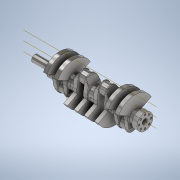
# Autodesk Inventor part: crankshaft
Saved by Autodesk Inventor 2021 (Build 250183000, 183)
## iProperties
Created: 2020-10-10
Part Number: crankshaft
Material: Сталь, высокопрочная, низколегированная
Document SubType Name: Modeling
Designer: panda
Density: 7.85 g/cm^3
Appearance: Сталь — полированная
Mass: 25968.1 g
Surface Area: 3777.36 cm^2
Volume: 3308.04 cm^3
Author: panda
Autodesk Inventor part; units mm, degrees
ref_plane "YZ Plane" through (0, 0, 0) normal (1, 0, 0) x (0, 1, 0)
ref_plane "XZ Plane" through (0, 0, 0) normal (0, 1, 0) x (-1, 0, 0)
ref_plane "XY Plane" through (0, 0, 0) normal (0, 0, 1) x (1, 0, 0)
sketch "Эскиз1" plane through (0, 0, 0) normal (1, 0, 0) x (0, 1, 0)
  circle A0 centre (0, 0) radius 27
  dimension "d0" = 54
  constraints: 1 centre point, 1 coincident
  measures "d0" diameter of A0
extrude "Выдавливание1" add sketch "Эскиз1" along normal blind 16.5
ref_plane "РабПлоскость1" through (36.5, 0, 0) normal (1, 0, 0) x (0, 0, -1)
sketch "Эскиз2" plane through (36.5, 0, 0) normal (1, 0, 0) x (0, 0, -1)
  circle A0 centre (0, 47.75) radius 33.9
  point P0 (0, 0)
  dimension "d4" = 67.8
  dimension "d5" = 47.75
  constraints: 1 centre point
  measures "d4" diameter of A0
  measures "d5" distance of point (0, 0) A0.centre
extrude "Выдавливание2" add sketch "Эскиз2" along normal blind 15.5
sketch "Эскиз3" plane through (36.5, 47.75, 0) normal (-1, 0, 0) x (0, 0, 1)
  circle A0 centre (0, 0) radius 33.9 projected
  arc A1 (-29.6851, -52.0851) -> (29.6851, -52.0851) centre (0, -47.75) ccw
  circle A2 centre (0, -47.75) radius 27 projected
  line L0 (36.5127, -5.3321) -> (29.6851, -52.0851)
  line L1 (-36.5127, -5.3321) -> (-29.6851, -52.0851)
  arc A3 (36.5127, -5.3321) -> (-36.5127, -5.3321) centre (0, 0) ccw
  dimension "d11" = 3
  dimension "d12" = 3
  constraints: 4 end point, 4 point on circle, 4 tangent, 2 centre point, 2 coincident
  measures "d11" radial gap between concentric circles of A1 A2
  measures "d12" radial gap between concentric circles of A3 A0
extrude "Выдавливание3" add sketch "Эскиз3" along normal up to surface (20 mm away) contours A0 A2 | A2 A0 | A0 A2 | L1 A3 L0 A1
sketch "Эскиз15" plane through (36.5, 47.75, 0) normal (1, 0, 0) x (0, 0, -1)
  arc A0 (0, 94) -> (-83.379, 43.4044) centre (0, 0) ccw
  line L0 (-83.379, 43.4044) -> (0, 0)
  line L1 (0, -114.4319) -> (0, 142.3414) projected
  arc A1 (83.379, 43.4044) -> (0, 94) centre (0, 0) ccw
  line L2 (83.379, 43.4044) -> (0, 0)
  arc A2 (36.5127, -5.3321) -> (-36.5127, -5.3321) centre (0, 0) ccw projected
  arc A3 (32.7307, 17.0385) -> (-32.7307, 17.0385) centre (0, 0) ccw
  point P0 (0, -47.75)
  dimension "d66" = 94
  dimension "d67" = 62.5
  constraints: 8 point on circle, 4 end point, 3 centre point, 2 point on line, 1 coincident, 1 symmetric about line, 1 other
  measures "d66" radius of A0
  measures "d67" angle of L0 L1
extrude "Выдавливание10" add sketch "Эскиз15" against normal up to surface (20 mm away) contours L1 A2 L0 A0 | A1 L2 A2 L1
fillet "Сопряжение3" radius 2 2 edges at (36.5, 47.75, 33.9) (16.5, -27, 0)
sketch "Эскиз4" plane through (0, 0, 0) normal (0, 0, 1) x (1, 0, 0)
  line L0 (16.5, 31.9847) -> (31.5, 78.15)
  line L1 (31.5, 78.15) -> (31.5, 84.65)
  line L2 (36.5, 84.65) -> (16.5, 84.65) projected
  line L3 (31.5, 84.65) -> (31.0691, 84.65)
  line L4 (36.5, 84.65) -> (36.5, 42.4179) projected
  line L5 (16.5, 84.65) -> (16.5, 42.4179) projected
  line L6 (16.5, 84.65) -> (16.5, 31.9847)
  line L7 (36.5, -30) -> (16.5, -30) projected
  line L8 (21.5, -30) -> (21.5, -21)
  line L9 (21.5, -21) -> (36.5, 4.9808)
  line L10 (36.5, 4.9808) -> (36.5, -30)
  line L11 (36.5, -30) -> (21.5, -30)
  line L12 (16.5, -4.3351) -> (16.5, -30) projected
  point P0 (0, 0)
  dimension "d23" = 5
  dimension "d24" = 6.5
  dimension "d25" = 72
  dimension "d26" = 60
  dimension "d27" = 5
  dimension "d28" = 9
  constraints: 16 end point, 3 point on line, 2 vertical, 1 horizontal, 1 parallel, 1 perpendicular
  measures "d23" distance from line of L4 L1.end
  measures "d24" distance of L0.end L1.end
  measures "d25" angle of L2 L0
  measures "d26" angle of L7 L9
  measures "d27" distance from line of L12 L8.start
  measures "d28" distance of L8.start L8.end
extrude "Выдавливание5" cut sketch "Эскиз4" along normal through all both and the other way through all contours L7 L8 L9 L10
fillet "Сопряжение4" radius 2 5 edges at (25.9318, -13.3239, 26.8789) (33.8107, 0.3228, 30.3654) (21.5, -30, 0) (25.9318, -13.3239, -26.8789) (33.8107, 0.3228, -30.3654)
mirror "Зеркальное отражение1" about plane through (52, 47.75, 0) normal (1, 0, 0) bodies 1 separate body
move or copy body "Переместить тело1" bodies to move or copy 2 copy no rotation origin (0, 0, 0) rotation axis (1, 0, 0) rotation angle 180 translate (0, 95.5, 0)
mirror "Зеркальное отражение2" about plane through (104, 95.5, 0) normal (1, 0, 0) bodies 2
mirror "Зеркальное отражение3" about plane through (0, 0, 0) normal (-1, 0, 0) of "Выдавливание1", "Выдавливание5", "Выдавливание3" bodies 1
mirror "Зеркальное отражение4" about plane through (156, 47.75, 0) normal (1, 0, 0) bodies 1 2
sketch "Эскиз7" plane through (348.5, 47.75, 0) normal (1, 0, 0) x (0, 0, -1)
  circle A0 centre (0, 0) radius 30.5
  point P0 (0, -47.75)
  dimension "d32" = 61
  constraints: 1 centre point
  measures "d32" diameter of A0
extrude "Выдавливание6" add sketch "Эскиз7" along normal blind 25 bodies 1
sketch "Эскиз8" plane through (373.5, 47.75, 0) normal (1, 0, 0) x (0, 0, -1)
  circle A0 centre (0, 0) radius 41
  point P0 (0, -47.75)
  dimension "d35" = 82
  constraints: 1 centre point
  measures "d35" diameter of A0
extrude "Выдавливание7" add sketch "Эскиз8" along normal blind 26 bodies 1
sketch "Эскиз9" plane through (-36.5, 47.75, 0) normal (-1, 0, 0) x (0, 0, 1)
  circle A0 centre (0, 0) radius 36
  point P0 (0, -47.75)
  dimension "d40" = 72
  constraints: 1 centre point
  measures "d40" diameter of A0
extrude "Выдавливание8" add sketch "Эскиз9" along normal blind 31 bodies 1
sketch "Эскиз10" plane through (-67.5, 47.75, 0) normal (-1, 0, 0) x (0, 0, 1)
  circle A0 centre (0, 0) radius 18
  point P0 (0, -47.75)
  dimension "d43" = 36
  constraints: 1 centre point
  measures "d43" diameter of A0
extrude "Выдавливание9" add sketch "Эскиз10" along normal blind 95 bodies 1
sketch "Эскиз11" plane through (-162.5, 47.75, 0) normal (-1, 0, 0) x (0, 0, 1)
  point P0 (0, -47.75)
  point P1 (0, 0)
hole "Отверстие1" at (-162.5, 47.75, 0) direction (1, 0, 0) diameter 17 depth 31 tip angle 118 countersink diameter 20 countersink angle 82 bodies 1
sketch "Эскиз13" plane through (0, 0, 0) normal (0, 0, 1) x (1, 0, 0)
  line L0 (-162.5, 39.4) -> (-162.5, 56.1) projected
  line L1 (52, 13.85) -> (52, 81.65) projected
  line L2 (260, 13.85) -> (260, 81.65) projected
  line L3 (89.5, 68.5) -> (118.5, 68.5) projected
  line L4 (89.5, 122.5) -> (118.5, 122.5) projected
  line L5 (193.5, 68.5) -> (222.5, 68.5) projected
  point P0 (0, 0)
  point P1 (52, 47.75)
  point P2 (-52, 47.75)
  point P3 (156, 47.75)
  point P4 (260, 47.75)
  constraints: 2 midpoint
hole "Отверстие2" at (156, 47.75, 0) at (52, 47.75, 0) at (260, 47.75, 0) at (-52, 47.75, 0) direction (0, 0, -1) diameter 7 end through all both bodies 1 2
sketch "Эскиз16" plane through (-36.5, 47.75, 0) normal (-1, 0, 0) x (0, 0, 1)
  arc A0 (83.379, 43.4044) -> (-83.379, 43.4044) centre (0, 0) ccw projected
  arc A1 (83.379, 43.4044) -> (-83.379, 43.4044) centre (0, 0) ccw
  arc A2 (36.5127, -5.3321) -> (32.7307, 17.0385) centre (0, 0) ccw projected
  arc A3 (-32.7307, 17.0385) -> (-36.5127, -5.3321) centre (0, 0) ccw projected
  arc A4 (32.7307, 17.0385) -> (-32.7307, 17.0385) centre (0, 0) ccw
  line L0 (-83.379, 43.4044) -> (0, 0)
  line L1 (0, 0) -> (83.379, 43.4044)
  point P0 (0, -47.75)
  point P1 (32.7307, 17.0385)
  point P2 (-83.379, 43.4044)
  constraints: 4 end point, 4 point on circle, 2 centre point, 1 coincident
extrude "Выдавливание11" add sketch "Эскиз16" against normal up to surface (20 mm away) contours L1 A4 L0 A0 bodies 1
sketch "Эскиз17" plane through (348.5, 47.75, 0) normal (1, 0, 0) x (0, 0, -1)
  line L0 (-83.379, 43.4044) -> (-32.7307, 17.0385) projected
  arc A0 (83.3727, 43.4166) -> (-83.379, 43.4044) centre (0, 0) ccw
  line L1 (-83.379, 43.4044) -> (0, 0)
  line L2 (0, 0) -> (83.3727, 43.4166)
  arc A1 (-36.5127, 5.3321) -> (-32.7307, -17.0385) centre (0, 0) ccw projected
  arc A2 (36.5127, -5.3321) -> (-36.5127, -5.3321) centre (0, 0) ccw projected
  arc A3 (32.7282, 17.0433) -> (-32.7307, 17.0385) centre (0, 0) ccw
  point P0 (0, -47.75)
  constraints: 5 point on circle, 4 end point, 2 centre point, 1 coincident, 1 point on line
extrude "Выдавливание12" add sketch "Эскиз17" against normal up to surface (20 mm away) contours A0 L2 A2 L0 bodies 1
move or copy body "Переместить тело2" bodies to move or copy 1 2 copy no translate (0, -47.75, 0)
sketch "Эскиз18" plane through (399.5, 0, 0) normal (1, 0, 0) x (0, 0, -1)
  point P0 (0, 0)
  point P1 (0, 0)
  constraints: 1 coincident
hole "Отверстие3" at (399.5, 0, 0) direction (-1, 0, 0) diameter 22.6568 depth 35 tip angle 118 countersink diameter 28 countersink angle 90 bodies 1 thread size "1-10 UNS" class "2B" standard "ANSI Unified Screw Threads"
sketch "Эскиз19" plane through (399.5, 0, 0) normal (1, 0, 0) x (0, 0, -1)
  circle A0 centre (0, 0) radius 30
  circle A1 centre (0, 0) radius 30.5 projected
  circle A2 centre (0, 0) radius 30
  circle A3 centre (0, 0) radius 30
  circle A4 centre (0, 0) radius 30
  circle A5 centre (0, 0) radius 30
  circle A6 centre (0, 0) radius 30
  circle A7 centre (0, 0) radius 30
  circle A8 centre (0, 0) radius 30
  point P0 (0, 30.5)
  point P1 (-21.5668, 21.5668)
  point P2 (-30.5, 0)
  point P3 (-21.5668, -21.5668)
  point P4 (0, -30.5)
  point P5 (21.5668, -21.5668)
  point P6 (30.5, 0)
  point P7 (21.5668, 21.5668)
  dimension "d86" = 60
  dimension "d89" = 360
  constraints: 8 centre point, 1 coincident, 1 vertical alignment, 26 other
  measures "d86" diameter of A0
hole "Отверстие4" at (399.5, 30.5, 0) at (399.5, 21.5668, 21.5668) at (399.5, 0, 30.5) at (399.5, -21.5668, 21.5668) at (399.5, -30.5, 0) at (399.5, -21.5668, -21.5668) at (399.5, 0, -30.5) at (399.5, 21.5668, -21.5668) direction (-1, 0, 0) diameter 7.7978 depth 15 tip angle 118 countersink diameter 10 countersink angle 90 bodies 1 thread size "3/8-16 UNC" class "2B" standard "ANSI Unified Screw Threads"
